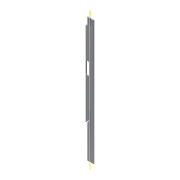
# Autodesk Inventor part: Horn support
Saved by Autodesk Inventor 2015 (Build 190159000, 159)
## iProperties
Created: 2016-04-07
Part Number: Horn support
Material: Generic
Document SubType Name: Modeling
Designer: jad211
Density: 1 g/cm^3
Appearance: Aluminum - Flat
Author: jad211
Autodesk Inventor part; units mm, degrees
ref_plane "YZ Plane" through (0, 0, 0) normal (1, 0, 0) x (0, 1, 0)
ref_plane "XZ Plane" through (0, 0, 0) normal (0, 1, 0) x (-1, 0, 0)
ref_plane "XY Plane" through (0, 0, 0) normal (0, 0, 1) x (1, 0, 0)
sketch "Sketch1" plane through (0, 0, 0) normal (0, 1, 0) x (-1, 0, 0)
  line L0 (0, 0) -> (25.4, 0)
  line L1 (25.4, 0) -> (25.4, -398)
  line L2 (25.4, -398) -> (0, -398)
  line L3 (0, -398) -> (0, 0)
  circle A0 centre (9.309, -142) radius 1.05
  line L4 (14.309, -132) -> (24.309, -132)
  line L5 (24.309, -132) -> (24.309, -152)
  line L6 (24.309, -152) -> (14.309, -152)
  line L7 (14.309, -152) -> (14.309, -132)
  line L8 (12.7, 0) -> (12.7, -398) construction
  dimension "d0" = 398
  dimension "d4" = 142
  dimension "d5" = 2.1
  dimension "d10" = 10
  dimension "d11" = 10
  dimension "d12" = 5
  dimension "d13" = 10
  dimension "d74" = 12.7
  dimension "d76" = 3.391
  constraints: 18 end point, 4 parallel, 2 horizontal, 2 midpoint, 2 perpendicular, 1 centre point
  measures "d0" distance of L0.end L1.end
  measures "d4" distance from line of L0 A0.centre
  measures "d5" diameter of A0
  measures "d10" distance from line of L6 A0.centre
  measures "d11" distance from line of L4 A0.centre
  measures "d12" distance from line of L7 A0.centre
  measures "d13" distance of L5.end L6.end
  measures "d74" distance between parallel lines of L3 L8
  measures "d76" distance from line of A0.centre L8
extrude "Extrusion2" add sketch "Sketch1" along normal blind 3.175 contours L0 L1 L2 L3 | L4 L5 L6 L7
ref_plane "Work Plane1" through (-12.7, 0, 0) normal (1, 0, 0) x (0, 0, -1)
sketch "Sketch2" plane through (0, 3.175, 0) normal (0, 1, 0) x (1, 0, 0)
  line L0 (-16.309, 122) -> (-22.309, 122)
  line L1 (-24.309, 124) -> (-24.309, 160)
  line L2 (-22.309, 162) -> (-16.309, 162)
  line L3 (-14.309, 160) -> (-14.309, 124)
  circle A0 centre (-9.309, 142) radius 1.05 projected
  arc A1 (-10.8091, 256) -> (-7.8091, 256) centre (-9.3091, 256) ccw
  line L4 (0, 398) -> (-25.4, 398) projected
  line L5 (0, 0) -> (0, 398) projected
  line L6 (-10.8091, 256) -> (-10.8091, 398)
  line L7 (-10.8091, 398) -> (-7.8091, 398)
  line L8 (-7.8091, 398) -> (-7.8091, 256)
  arc A2 (-17.1409, 256) -> (-15.0409, 256) centre (-16.0909, 256) ccw
  line L9 (-15.0409, 256) -> (-15.0409, 286.2615)
  line L10 (-17.1409, 285.4641) -> (-17.1409, 256)
  line L11 (-17.6449, 286.7915) -> (-23.7779, 293.7031)
  line L12 (-25.7091, 294.203) -> (-25.7091, 398)
  line L13 (-15.5449, 287.5889) -> (-19.2051, 291.7137)
  line L14 (-19.7091, 293.0412) -> (-19.7091, 398)
  line L15 (-25.7091, 398) -> (-19.7091, 398)
  line L16 (-25.4, 0) -> (0, 0) projected
  line L17 (-7.8091, 0) -> (-10.8091, 0)
  line L18 (-10.8091, 0) -> (-10.8091, 23.5)
  line L19 (-7.8091, 23.5) -> (-7.8091, 0)
  line L20 (-19.7091, 0) -> (-25.7091, 0)
  line L21 (-25.7091, 0) -> (-25.7091, 25)
  line L22 (-19.7091, 23) -> (-19.7091, 0)
  arc A3 (-22.309, 162) -> (-24.309, 160) centre (-22.309, 160) ccw
  arc A4 (-14.309, 160) -> (-16.309, 162) centre (-16.309, 160) ccw
  arc A5 (-24.309, 124) -> (-22.309, 122) centre (-22.309, 124) ccw
  arc A6 (-16.309, 122) -> (-14.309, 124) centre (-16.309, 124) ccw
  arc A7 (-19.7091, 293.0412) -> (-19.2051, 291.7137) centre (-17.7091, 293.0412) ccw
  arc A8 (-17.1409, 285.4641) -> (-17.6449, 286.7915) centre (-19.1409, 285.4641) ccw
  arc A9 (-15.0409, 286.2615) -> (-15.5449, 287.5889) centre (-17.0409, 286.2615) ccw
  circle A10 centre (-15.7, 7) radius 1.5
  line L23 (-25.4, 0) -> (-25.4, 398) projected
  arc A11 (-7.8091, 23.5) -> (-10.8091, 23.5) centre (-9.3091, 23.5) ccw
  line L24 (-12.7, 398) -> (-12.7, 0) construction
  line L25 (-22.7091, 398) -> (-22.7091, 316.511) construction
  line L26 (-21.7091, 25) -> (-25.7091, 25)
  arc A12 (-19.7091, 23) -> (-21.7091, 25) centre (-21.7091, 23) ccw
  circle A13 centre (-3.7, 7) radius 1.5
  line L27 (-25.7091, 296.4624) -> (-25.7091, 292.6371)
  line L28 (-25.7091, 292.6371) -> (-25.7091, 288.9391)
  line L29 (-25.7091, 288.9391) -> (-25.4, 288.9391)
  line L30 (-25.4, 398) -> (-25.4, 0) projected
  line L31 (-25.4, 292.9202) -> (-25.4, 288.9391)
  arc A14 (-23.7779, 293.7031) -> (-25.4, 292.9202) centre (-24.4, 292.9202) ccw
  circle A15 centre (-15.7, 14) radius 1.5
  circle A16 centre (-3.7, 14) radius 1.5
  point P0 (-14.309, 122)
  point P1 (-24.309, 162)
  point P2 (-24.309, 122)
  point P3 (-14.309, 162)
  point P4 (-15.0409, 287.0209)
  point P5 (-17.1409, 286.2235)
  point P6 (-25.7091, 295.8795)
  point P7 (-19.7091, 292.2818)
  dimension "d14" = 5
  dimension "d15" = 10
  dimension "d16" = 40
  dimension "d17" = 20
  dimension "d25" = 6.7818
  dimension "d45" = 2
  dimension "d83" = 25.4
  dimension "d84" = 9.309
  dimension "d87" = 3
  dimension "d89" = 3
  dimension "d90" = 6
  dimension "d91" = 2.1
  dimension "d92" = 2.1
  dimension "d93" = 1.05
  dimension "d94" = 1.5
  dimension "d95" = 12.7
  dimension "d97" = 3.3909
  dimension "d98" = 13.4
  dimension "d99" = 3
  dimension "d100" = 3.3909
  dimension "d105" = 1.5
  dimension "d107" = 2
  dimension "d111" = 7
  dimension "d114" = 8.9
  dimension "d116" = 6
  dimension "d117" = 0
  dimension "d120" = 3
  dimension "d123" = 3
  dimension "d124" = 9
  dimension "d127" = 1
  dimension "d129" = 7
  dimension "d130" = 7
  dimension "d131" = 0
  dimension "d132" = 3
  dimension "d133" = 3
  dimension "d134" = 7
  dimension "d135" = 9
  dimension "d144" = 25
  dimension "d145" = 23.5
  constraints: 54 end point, 24 point on circle, 24 point on line, 16 centre point, 16 tangent, 10 parallel, 6 equal radius, 6 perpendicular, 5 horizontal, 3 midpoint, 1 collinear, 1 vertical
  measures "d14" distance from line of L3 A0.centre
  measures "d15" distance of point (-24.309, 162) point (-14.309, 162)
  measures "d16" distance of point (-24.309, 122) point (-24.309, 162)
  measures "d17" distance from line of L2 A0.centre
  measures "d25" distance of A1.centre A2.centre
  measures "d45" radius of A3
  measures "d83" distance between parallel lines of L23 L5
  measures "d84" distance from line of L5 A0.centre
  measures "d87" diameter of A10
  measures "d89" distance between parallel lines of L6 L8
  measures "d90" distance between parallel lines of L12 L14
  measures "d91" distance between parallel lines of L11 L13
  measures "d92" distance between parallel lines of L10 L9
  measures "d93" radius of A2
  measures "d94" radius of A1
  measures "d95" distance between parallel lines of L23 L24
  measures "d97" distance from line of L24 A1.centre
  measures "d98" distance from line of L25 A1.centre
  measures "d99" distance between parallel lines of L18 L19
  measures "d100" distance from line of L24 A11.centre
  measures "d105" radius of A11
  measures "d107" radius of A12
  measures "d111" distance from line of L16 A10.centre
  measures "d114" distance between parallel lines of L6 L14
  measures "d116" distance between parallel lines of L21 L22
  measures "d117" distance between parallel lines of L14 L22
  measures "d120" diameter of A13
  measures "d123" distance from line of L24 A10.centre
  measures "d124" distance from line of L24 A13.centre
  measures "d127" radius of A14
  measures "d129" distance from line of L16 A13.centre
  measures "d130" distance of A15.centre A10.centre
  measures "d131" horizontal distance of A10.centre A15.centre
  measures "d132" diameter of A15
  measures "d133" diameter of A16
  measures "d134" distance of A16.centre A13.centre
  measures "d135" distance from line of L24 A16.centre
  measures "d144" distance between parallel lines of L16 L26
  measures "d145" distance from line of L16 A11.centre
extrude "Extrusion8" cut sketch "Sketch2" against normal up to next contours L0 A5 L1 A3 L2 A4 L3 A6 | L6 L4 L8 A1 | L14 A7 L13 A9 L9 A2 L10 A8 L11 A14 L23 L4 | L23 L29 L28 L27 L12 L15 | L16 L18 A11 L19 | L26 A12 L22 L16 L23 | L23 L20 L21 L26 | A10 | A13 | A15 | A16
thread "Thread1" size "M3x0.5" class "6H" standard "ANSI Metric M Profile" full length
thread "Thread2" size "M3x0.5" class "6H" standard "ANSI Metric M Profile" full length
thread "Thread3" size "M3x0.5" class "6H" standard "ANSI Metric M Profile" full length
thread "Thread4" size "M3x0.5" class "6H" standard "ANSI Metric M Profile" full length
thread "Thread5" size "M2.2x0.45" class "6H" standard "ANSI Metric M Profile" full length
equation "\"d95\" = 0.5 * d83"
equation "\"d97\" = 0.5 * d25"
equation "\"d99\" = d89"
equation "\"d100\" = d97"
equation "\"d105\" = 0.5 * d99"
equation "\"d116\" = d90"
equation "\"d120\" = d87"
equation "\"d125\" = d120"
body "Solid2"
